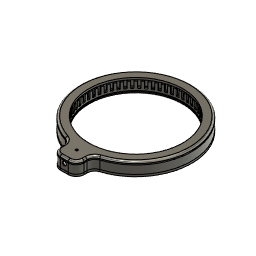
chassis_router (Autodesk Fusion 360 design; units mm, degrees)
Autodesk Fusion 360 part; units mm, degrees
ref_plane "WorkPlane1" through (0, 3.302, 0) normal (0, 1, 0) x (0, 0, 1)
sketch "l1_mirror_base" plane through (0, 0, 0) normal (0, 1, 0) x (1, 0, 0)
  circle A0 centre (0, 0) radius 180.975
  circle A1 centre (0, 0) radius 152.4
  line L0 (0, 0) -> (-90.4875, 156.7289) construction
  line L1 (0, 0) -> (0, 180.975) construction
  circle A2 centre (-84.455, 146.2804) radius 4.445
  line L2 (-84.455, 146.2804) -> (-88.9, 146.2804) construction
  line L3 (-84.455, 146.2804) -> (-80.01, 146.2804) construction
  line L4 (-86.36, 150.2964) -> (-82.55, 150.2964)
  line L5 (86.36, 150.2964) -> (82.55, 150.2964)
  line L6 (84.455, 146.2804) -> (80.01, 146.2804) construction
  circle A3 centre (84.455, 146.2804) radius 4.445
  line L7 (84.455, 146.2804) -> (88.9, 146.2804) construction
  line L8 (0, 0) -> (0, -180.975) construction
  line L9 (-38.1, -176.919) -> (38.1, -176.919)
  line L10 (38.1, -176.919) -> (38.1, -206.129)
  line L11 (12.7, -231.529) -> (-12.7, -231.529)
  line L12 (-38.1, -206.129) -> (-38.1, -176.919)
  arc A4 (12.7, -231.529) -> (38.1, -206.129) centre (12.7, -206.129) ccw
  arc A5 (-38.1, -206.129) -> (-12.7, -231.529) centre (-12.7, -206.129) ccw
  line L13 (34.925, -185.809) -> (34.925, -206.129)
  arc A6 (12.7, -228.354) -> (34.925, -206.129) centre (12.7, -206.129) ccw
  line L14 (12.7, -228.354) -> (-12.7, -228.354)
  arc A7 (-34.925, -206.129) -> (-12.7, -228.354) centre (-12.7, -206.129) ccw
  line L15 (-34.925, -206.129) -> (-34.925, -185.809)
  line L16 (-28.575, -179.459) -> (28.575, -179.459)
  arc A8 (-28.575, -179.459) -> (-34.925, -185.809) centre (-28.575, -185.809) ccw
  arc A9 (34.925, -185.809) -> (28.575, -179.459) centre (28.575, -185.809) ccw
  arc A10 (-38.1, -196.3629) -> (-55.6846, -172.1952) centre (-63.5, -196.3629) ccw
  arc A11 (55.6846, -172.1952) -> (38.1, -196.3629) centre (63.5, -196.3629) ccw
  line L17 (-84.455, 146.2804) -> (-84.455, 150.2964) construction
  line L18 (-82.55, 150.2964) -> (-82.55, 155.3764)
  line L19 (-86.36, 150.2964) -> (-86.36, 155.3764)
  arc A12 (-82.55, 155.3764) -> (-86.36, 155.3764) centre (-84.455, 155.3764) ccw
  line L20 (-82.55, 155.3764) -> (-86.36, 155.3764) construction
  line L21 (86.36, 150.2964) -> (86.36, 155.3764)
  line L22 (82.55, 150.2964) -> (82.55, 155.3764)
  arc A13 (86.36, 155.3764) -> (82.55, 155.3764) centre (84.455, 155.3764) ccw
  line L23 (86.36, 155.3764) -> (82.55, 155.3764)
  point P0 (90.4875, 156.7289)
  point P1 (38.1, -231.529)
  point P2 (-38.1, -231.529)
  dimension "d12" = 361.95
  dimension "d16" = 304.8
  dimension "d85" = 30
  dimension "d91" = 168.91
  dimension "d99" = 8.89
  dimension "d52" = 76.2
  dimension "d54" = 54.61
  dimension "d55" = 25.4
  dimension "d56" = 25.4
  dimension "d58" = 6.35
  dimension "d59" = 3.175
  dimension "d60" = 2.54
  dimension "d61" = 25.4
  dimension "d141" = 3.81
  dimension "d142" = 5.08
  dimension "d143" = 5.08
  constraint coincident A0.centre A1.centre
  constraint coincident A0 L0.end
  constraint coincident A0 L1.end
  constraint vertical L1
  constraint coincident L0 A2.centre
  constraint coincident A2.centre L2.start
  constraint coincident A2 L2.end
  constraint coincident A2 L3.end
  constraint parallel L2 L3
  constraint horizontal L4
  constraint coincident A2 L4.end
  constraint horizontal L2
  constraint symmetric L0.end L1 P0
  constraint symmetric L1 A2 A3
  constraint symmetric L1 A2.centre L6.start
  constraint symmetric L1 L2.end L7.end
  constraint symmetric L1 L3.end L6.end
  constraint symmetric L1 L4.start L5.start
  constraint symmetric L1 L4.end L5.end
  constraint coincident A0 L8.end
  constraint parallel L1 L8
  constraint horizontal L9
  constraint vertical L10
  constraint horizontal L11
  constraint vertical L12
  constraint coincident A0 L9.start
  constraint coincident P1 L10
  constraint coincident P1 L11
  constraint tangent L10 A4
  constraint tangent L11 A4
  constraint coincident P2 L11
  constraint coincident P2 L12
  constraint tangent L11 A5
  constraint tangent L12 A5
  constraint parallel L10 L13
  constraint concentric A4 A6
  constraint parallel L11 L14
  constraint concentric A5 A7
  constraint parallel L12 L15
  constraint parallel L9 L16
  constraint tangent L13 A6
  constraint tangent A6 L14
  constraint tangent L14 A7
  constraint tangent A7 L15
  constraint tangent L16 A8
  constraint tangent L15 A8
  constraint tangent L13 A9
  constraint tangent L16 A9
  constraint equal A8 A9
  constraint tangent A0 A10
  constraint coincident A0 A10.end
  constraint coincident L12 A10.start
  constraint tangent L12 A10
  constraint symmetric L8 A10.end A11.start
  constraint symmetric L8 A10.start A11.end
  constraint symmetric L8 A10 A11
  constraint midpoint L4 L17.end
  constraint perpendicular L4 L17
  constraint perpendicular L4 L18
  constraint perpendicular L4 L19
  constraint equal L18 L19
  constraint coincident A12.centre L20
  constraint perpendicular L5 L21
  constraint perpendicular L5 L22
  constraint equal L21 L22
  constraint coincident A13.centre L23
  measures "d12" diameter of A0
  measures "d16" diameter of A1
  measures "d85" angle of L0 L1
  measures "d91" distance of A0.centre A2.centre
  measures "d99" diameter of A2
  measures "d52" distance of P1 P2
  measures "d54" distance of L9.end P1
  measures "d55" radius of A4
  measures "d56" radius of A5
  measures "d58" radius of A8
  measures "d59" distance of L12 L15
  measures "d60" distance of L9 L16
  measures "d61" radius of A10
  measures "d141" distance of L4.start L4.end
  measures "d142" distance of L4.end L18.end
  measures "d143" distance of L5.end L22.end
extrude "Extrude1" add sketch "l1_mirror_base" along normal up to surface (3.302 mm away) contours A0 L9 | A0 L12 A10 | A0 L10 A11 | A0 L9 L16 | A0 L10 L11 L12 A4 A5 L13 A6 L14 A7 L15 L16 A8 A9 | A0 L16 makes body 1
ref_plane "WorkPlane2" through (0, 6.35, 0) normal (0, 1, 0) x (0, 0, 1)
sketch "l1_mirror" plane through (0, 3.302, 0) normal (0, 1, 0) x (1, 0, 0)
  circle A0 centre (0, 0) radius 180.975
  circle A1 centre (0, 0) radius 163.195
  circle A2 centre (-84.455, 146.2804) radius 4.445
  circle A3 centre (84.455, 146.2804) radius 4.445
  arc A4 (55.6846, -172.1952) -> (-55.6846, -172.1952) centre (0, 0) ccw
  line L0 (-38.1, -196.3629) -> (-38.1, -206.129)
  arc A5 (-38.1, -206.129) -> (-12.7, -231.529) centre (-12.7, -206.129) ccw
  line L1 (-12.7, -231.529) -> (12.7, -231.529)
  arc A6 (12.7, -231.529) -> (38.1, -206.129) centre (12.7, -206.129) ccw
  line L2 (38.1, -206.129) -> (38.1, -196.3629)
  line L3 (-28.575, -179.459) -> (-23.3754, -179.459)
  line L4 (34.925, -185.809) -> (34.925, -206.129)
  arc A7 (12.7, -228.354) -> (34.925, -206.129) centre (12.7, -206.129) ccw
  line L5 (12.7, -228.354) -> (-12.7, -228.354)
  arc A8 (-34.925, -206.129) -> (-12.7, -228.354) centre (-12.7, -206.129) ccw
  line L6 (-34.925, -206.129) -> (-34.925, -185.809)
  arc A9 (-28.575, -179.459) -> (-34.925, -185.809) centre (-28.575, -185.809) ccw
  arc A10 (34.925, -185.809) -> (28.575, -179.459) centre (28.575, -185.809) ccw
  arc A11 (-38.1, -196.3629) -> (-55.6846, -172.1952) centre (-63.5, -196.3629) ccw
  arc A12 (55.6846, -172.1952) -> (38.1, -196.3629) centre (63.5, -196.3629) ccw
  arc A13 (-23.3754, -179.459) -> (23.3754, -179.459) centre (0, 0) ccw
  line L7 (23.3754, -179.459) -> (28.575, -179.459)
  circle A14 centre (0, 0) radius 152.4
  line L8 (-82.55, 155.3764) -> (-82.55, 150.2964)
  arc A15 (-86.36, 150.2964) -> (-82.55, 150.2964) centre (-84.455, 146.2804) ccw
  line L9 (-86.36, 150.2964) -> (-86.36, 155.3764)
  arc A16 (-82.55, 155.3764) -> (-86.36, 155.3764) centre (-84.455, 155.3764) ccw
  line L10 (86.36, 155.3764) -> (86.36, 150.2964)
  arc A17 (82.55, 150.2964) -> (86.36, 150.2964) centre (84.455, 146.2804) ccw
  line L11 (82.55, 150.2964) -> (82.55, 155.3764)
  arc A18 (86.36, 155.3764) -> (82.55, 155.3764) centre (84.455, 155.3764) ccw
  arc A19 (-86.36, 150.2964) -> (-82.55, 150.2964) centre (-84.455, 146.2804) ccw
  line L12 (-82.55, 150.2964) -> (-82.55, 155.3764)
  arc A20 (-82.55, 155.3764) -> (-86.36, 155.3764) centre (-84.455, 155.3764) ccw
  line L13 (-86.36, 155.3764) -> (-86.36, 150.2964)
  arc A21 (82.55, 150.2964) -> (86.36, 150.2964) centre (84.455, 146.2804) ccw
  line L14 (86.36, 150.2964) -> (86.36, 155.3764)
  arc A22 (86.36, 155.3764) -> (82.55, 155.3764) centre (84.455, 155.3764) ccw
  line L15 (82.55, 155.3764) -> (82.55, 150.2964)
  circle A23 centre (0, 0) radius 152.4
  arc A24 (12.7, -228.354) -> (34.925, -206.129) centre (12.7, -206.129) ccw
  line L16 (34.925, -206.129) -> (34.925, -185.809)
  arc A25 (34.925, -185.809) -> (28.575, -179.459) centre (28.575, -185.809) ccw
  line L17 (28.575, -179.459) -> (23.3754, -179.459)
  arc A26 (-23.3754, -179.459) -> (23.3754, -179.459) centre (0, 0) ccw
  line L18 (-23.3754, -179.459) -> (-28.575, -179.459)
  arc A27 (-28.575, -179.459) -> (-34.925, -185.809) centre (-28.575, -185.809) ccw
  line L19 (-34.925, -185.809) -> (-34.925, -206.129)
  arc A28 (-34.925, -206.129) -> (-12.7, -228.354) centre (-12.7, -206.129) ccw
  line L20 (-12.7, -228.354) -> (12.7, -228.354)
  arc A29 (-38.1, -206.129) -> (-12.7, -231.529) centre (-12.7, -206.129) ccw
  line L21 (-38.1, -206.129) -> (-38.1, -196.3629)
  arc A30 (-38.1, -196.3629) -> (-55.6846, -172.1952) centre (-63.5, -196.3629) ccw
  arc A31 (55.6846, -172.1952) -> (-55.6846, -172.1952) centre (0, 0) ccw
  arc A32 (55.6846, -172.1952) -> (38.1, -196.3629) centre (63.5, -196.3629) ccw
  line L22 (38.1, -196.3629) -> (38.1, -206.129)
  arc A33 (12.7, -231.529) -> (38.1, -206.129) centre (12.7, -206.129) ccw
  line L23 (12.7, -231.529) -> (-12.7, -231.529)
  line L24 (84.455, 146.2804) -> (80.01, 146.2804) construction
  line L25 (84.455, 146.2804) -> (88.9, 146.2804) construction
  line L26 (88.9, 146.2804) -> (88.9, 152.8364)
  line L27 (80.01, 146.2804) -> (80.01, 152.8364)
  arc A34 (88.9, 152.8364) -> (80.01, 152.8364) centre (84.455, 152.8364) ccw
  line L28 (-84.455, 146.2804) -> (-88.9, 146.2804) construction
  line L29 (-84.455, 146.2804) -> (-80.01, 146.2804) construction
  line L30 (-80.01, 146.2804) -> (-80.01, 156.0262)
  line L31 (-88.9, 146.2804) -> (-88.9, 156.0262)
  line L32 (84.455, 146.2804) -> (84.455, 157.2814) construction
  line L33 (-84.455, 146.2804) -> (-84.455, 157.2814) construction
  circle A35 centre (-84.455, 152.8364) radius 4.445
  dimension "d18" = 361.95
  dimension "d19" = 326.39
  constraint coincident A0.centre A1.centre
  constraint coincident A3.centre A17.centre
  constraint coincident A21 L24.end
  constraint coincident A21 L25.end
  constraint tangent A21 L26
  constraint tangent A21 L27
  constraint tangent L27 A34
  constraint tangent L26 A34
  constraint coincident A2.centre A15.centre
  constraint coincident A19 L28.end
  constraint coincident A19 L29.end
  constraint tangent A15 L30
  constraint perpendicular L29 L30
  constraint tangent A2 L31
  constraint perpendicular L28 L31
  constraint midpoint A22 L32.end
  constraint perpendicular L24 L32
  constraint perpendicular L25 L32
  constraint tangent A22 A34
  constraint midpoint A16 L33.end
  constraint perpendicular L28 L33
  constraint perpendicular L29 L33
  constraint tangent A20 A35
  constraint tangent L30 A35
  constraint equal L30 L31
  constraint tangent L31 A35
  measures "d18" diameter of A0
  measures "d19" diameter of A1
extrude "Extrude2" add sketch "l1_mirror" along normal up to surface (3.048 mm away) contours A0 A4 A13 A26 A31 | A0 L0 A5 L1 A6 L2 L3 L4 A7 L5 A8 L6 A9 A10 A11 A12 L7 A24 L16 A25 L17 L18 A27 L19 A28 L20 A29 L21 A30 A32 L22 A33 L23 bodies 1
ref_plane "WorkPlane3" through (0, 14.097, 0) normal (0, 1, 0) x (0, 0, 1)
sketch "l2_led_base" plane through (0, 6.35, 0) normal (0, 1, 0) x (1, 0, 0)
  circle A0 centre (0, 0) radius 180.975
  circle A1 centre (0, 0) radius 152.4
  line L0 (0, 0) -> (-9.4715, 180.727) construction
  line L1 (0, 0) -> (0, 180.975) construction
  arc A2 (55.6846, -172.1952) -> (-55.6846, -172.1952) centre (0, 0) ccw
  arc A3 (-38.1, -196.3629) -> (-55.6846, -172.1952) centre (-63.5, -196.3629) ccw
  line L2 (-38.1, -196.3629) -> (-38.1, -206.129)
  arc A4 (-38.1, -206.129) -> (-12.7, -231.529) centre (-12.7, -206.129) ccw
  line L3 (-12.7, -231.529) -> (12.7, -231.529)
  arc A5 (12.7, -231.529) -> (38.1, -206.129) centre (12.7, -206.129) ccw
  line L4 (38.1, -206.129) -> (38.1, -196.3629)
  arc A6 (55.6846, -172.1952) -> (38.1, -196.3629) centre (63.5, -196.3629) ccw
  line L5 (88.9, 152.8364) -> (88.9, 146.2804)
  arc A7 (80.01, 146.2804) -> (88.9, 146.2804) centre (84.455, 146.2804) ccw
  line L6 (80.01, 146.2804) -> (80.01, 152.8364)
  arc A8 (88.9, 152.8364) -> (80.01, 152.8364) centre (84.455, 152.8364) ccw
  arc A9 (-28.575, -179.459) -> (-34.925, -185.809) centre (-28.575, -185.809) ccw
  line L7 (-28.575, -179.459) -> (-23.3754, -179.459)
  arc A10 (-23.3754, -179.459) -> (23.3754, -179.459) centre (0, 0) ccw
  line L8 (23.3754, -179.459) -> (28.575, -179.459)
  arc A11 (34.925, -185.809) -> (28.575, -179.459) centre (28.575, -185.809) ccw
  line L9 (34.925, -185.809) -> (34.925, -206.129)
  arc A12 (12.7, -228.354) -> (34.925, -206.129) centre (12.7, -206.129) ccw
  line L10 (12.7, -228.354) -> (-12.7, -228.354)
  arc A13 (-34.925, -206.129) -> (-12.7, -228.354) centre (-12.7, -206.129) ccw
  line L11 (-34.925, -206.129) -> (-34.925, -185.809)
  line L12 (-80.01, 152.8364) -> (-80.01, 146.2804)
  arc A14 (-88.9, 146.2804) -> (-80.01, 146.2804) centre (-84.455, 146.2804) ccw
  line L13 (-88.9, 146.2804) -> (-88.9, 152.8364)
  arc A15 (-80.01, 152.8364) -> (-88.9, 152.8364) centre (-84.455, 152.8364) ccw
  circle A16 centre (0, 0) radius 163.195
  dimension "d23" = 361.95
  dimension "d24" = 304.8
  dimension "d1" = 3
  constraint coincident A0.centre A1.centre
  constraint coincident A0 L0.end
  constraint coincident A0 L1.end
  constraint vertical L1
  measures "d23" diameter of A0
  measures "d24" diameter of A1
  measures "d1" angle of L0 L1
extrude "Extrude3" add sketch "l2_led_base" along normal up to surface (7.747 mm away) separate body contours A0 A2 A10 | A0 A3 L2 A4 L3 A5 L4 A6 A9 L7 L8 A11 L9 A12 L10 A13 L11 | L5 A7 L6 A8 | L12 A14 L13 A15 | A16 makes body 2
ref_plane "WorkPlane4" through (0, 32.8422, 0) normal (0, 1, 0) x (0, 0, 1)
sketch "l2_leds" plane through (0, 14.097, 0) normal (0, 1, 0) x (1, 0, 0)
  circle A0 centre (0, 0) radius 180.975
  circle A1 centre (0, 0) radius 159.639
  line L0 (0, 0) -> (0, 180.975) construction
  circle A2 centre (0, 0) radius 152.4 construction
  line L1 (0, 0) -> (-7.976, 152.1911) construction
  line L2 (0, 0) -> (-11.9572, 151.9302) construction
  line L3 (0, 0) -> (-3.9894, 152.3478) construction
  arc A3 (-3.9894, 152.3478) -> (-11.9572, 151.9302) centre (0, 0) ccw
  circle A4 centre (0, 0) radius 157.099
  line L4 (-3.9894, 152.3478) -> (4.1124, -157.0452)
  line L5 (-11.9572, 151.9302) -> (12.3258, -156.6147)
  line L6 (-3.9894, 152.3478) -> (-4.1124, 157.0452)
  line L7 (-11.9572, 151.9302) -> (-12.3258, 156.6147)
  arc A5 (55.6846, -172.1952) -> (38.1, -196.3629) centre (63.5, -196.3629) ccw
  arc A6 (-38.1, -196.3629) -> (-55.6846, -172.1952) centre (-63.5, -196.3629) ccw
  line L8 (-38.1, -196.3629) -> (-38.1, -206.129)
  arc A7 (-38.1, -206.129) -> (-12.7, -231.529) centre (-12.7, -206.129) ccw
  line L9 (-12.7, -231.529) -> (12.7, -231.529)
  arc A8 (12.7, -231.529) -> (38.1, -206.129) centre (12.7, -206.129) ccw
  line L10 (38.1, -206.129) -> (38.1, -196.3629)
  line L11 (0, 0) -> (0, -171.45) construction
  line L12 (6.35, -159.5127) -> (6.35, -180.8636)
  line L13 (-6.35, -180.8636) -> (-6.35, -159.5127)
  arc A9 (9.3393, -159.3656) -> (6.35, -162.5351) centre (9.525, -162.5351) ccw
  arc A10 (-6.35, -162.5351) -> (-9.3393, -159.3656) centre (-9.525, -162.5351) ccw
  circle A11 centre (0, 0) radius 152.4
  arc A12 (55.6846, -172.1952) -> (-55.6846, -172.1952) centre (0, 0) ccw
  arc A13 (55.6846, -172.1952) -> (38.1, -196.3629) centre (63.5, -196.3629) ccw
  arc A14 (55.6846, -172.1952) -> (-55.6846, -172.1952) centre (0, 0) ccw
  arc A15 (-38.1, -196.3629) -> (-55.6846, -172.1952) centre (-63.5, -196.3629) ccw
  line L14 (-38.1, -196.3629) -> (-38.1, -206.129)
  arc A16 (-38.1, -206.129) -> (-12.7, -231.529) centre (-12.7, -206.129) ccw
  line L15 (-12.7, -231.529) -> (12.7, -231.529)
  arc A17 (12.7, -231.529) -> (38.1, -206.129) centre (12.7, -206.129) ccw
  line L16 (38.1, -206.129) -> (38.1, -196.3629)
  line L17 (88.9, 152.8364) -> (88.9, 146.2804)
  arc A18 (80.01, 146.2804) -> (88.9, 146.2804) centre (84.455, 146.2804) ccw
  line L18 (80.01, 146.2804) -> (80.01, 152.8364)
  arc A19 (88.9, 152.8364) -> (80.01, 152.8364) centre (84.455, 152.8364) ccw
  arc A20 (-28.575, -179.459) -> (-34.925, -185.809) centre (-28.575, -185.809) ccw
  line L19 (-28.575, -179.459) -> (-23.3754, -179.459)
  arc A21 (-23.3754, -179.459) -> (23.3754, -179.459) centre (0, 0) ccw
  line L20 (23.3754, -179.459) -> (28.575, -179.459)
  arc A22 (34.925, -185.809) -> (28.575, -179.459) centre (28.575, -185.809) ccw
  line L21 (34.925, -185.809) -> (34.925, -206.129)
  arc A23 (12.7, -228.354) -> (34.925, -206.129) centre (12.7, -206.129) ccw
  line L22 (12.7, -228.354) -> (-12.7, -228.354)
  arc A24 (-34.925, -206.129) -> (-12.7, -228.354) centre (-12.7, -206.129) ccw
  line L23 (-34.925, -206.129) -> (-34.925, -185.809)
  line L24 (-80.01, 152.8364) -> (-80.01, 146.2804)
  arc A25 (-88.9, 146.2804) -> (-80.01, 146.2804) centre (-84.455, 146.2804) ccw
  line L25 (-88.9, 146.2804) -> (-88.9, 152.8364)
  arc A26 (-80.01, 152.8364) -> (-88.9, 152.8364) centre (-84.455, 152.8364) ccw
  circle A27 centre (0, 0) radius 163.195
  line L26 (34.925, -185.809) -> (34.925, -206.129)
  arc A28 (12.7, -228.354) -> (34.925, -206.129) centre (12.7, -206.129) ccw
  line L27 (12.7, -228.354) -> (-12.7, -228.354)
  arc A29 (-34.925, -206.129) -> (-12.7, -228.354) centre (-12.7, -206.129) ccw
  line L28 (-34.925, -206.129) -> (-34.925, -185.809)
  arc A30 (-28.575, -179.459) -> (-34.925, -185.809) centre (-28.575, -185.809) ccw
  line L29 (-28.575, -179.459) -> (-23.3754, -179.459)
  arc A31 (-23.3754, -179.459) -> (23.3754, -179.459) centre (0, 0) ccw
  line L30 (23.3754, -179.459) -> (28.575, -179.459)
  arc A32 (34.925, -185.809) -> (28.575, -179.459) centre (28.575, -185.809) ccw
  dimension "d28" = 361.95
  dimension "d29" = 319.278
  dimension "d6" = 304.8
  dimension "d7" = 3
  dimension "d8" = 3
  dimension "d10" = 314.198
  dimension "d100" = 12.7
  dimension "d101" = 3.175
  constraint coincident A0.centre A1.centre
  constraint concentric A0 A1
  constraint coincident A0 L0.end
  constraint vertical L0
  constraint coincident A2 L1.end
  constraint coincident A2 L2.end
  constraint coincident A2 L3.end
  constraint symmetric L1 L2 L3
  constraint concentric A2 A3
  constraint concentric A2 A4
  constraint coincident A4 L4.end
  constraint parallel L3 L4
  constraint coincident A4 L5.end
  constraint parallel L2 L5
  constraint coincident A4 L6.end
  constraint parallel L4 L6
  constraint coincident A4 L7.end
  constraint parallel L5 L7
  constraint coincident A1 L12.start
  constraint coincident A1 L13.end
  constraint vertical L13
  constraint vertical L12
  constraint symmetric L11 L12 L13
  constraint tangent A1 A9
  constraint coincident A1 A9.start
  constraint coincident L12 A9.end
  constraint tangent L12 A9
  constraint symmetric L11 A9.end A10.start
  constraint symmetric L11 A9.start A10.end
  constraint symmetric L11 A9 A10
  constraint coincident A0 L12.end
  constraint coincident A0 L13.start
  measures "d28" diameter of A0
  measures "d29" diameter of A1
  measures "d6" diameter of A2
  measures "d7" angle of L0 L1
  measures "d8" angle of L2 L3
  measures "d10" diameter of A4
  measures "d100" distance of L12 L13
  measures "d101" radius of A9
extrude "Extrude4" add sketch "l2_leds" along normal up to surface (18.7452 mm away) contours A0 L12 L13 A12 A14 A21 A27 A31 | A0 A5 A6 L8 A7 L9 A8 L10 A13 A15 L14 A16 L15 A17 L16 A20 L19 L20 A22 L21 A23 L22 A24 L23 L26 A28 L27 A29 L28 A30 L29 L30 A32 | A1 L12 L13 A9 A10 A27 | L17 A18 L18 A19 | L24 A25 L25 A26 bodies 2
sketch "l3_cap_base" plane through (0, 32.8422, 0) normal (0, 1, 0) x (1, 0, 0)
  circle A0 centre (0, 0) radius 180.975
  circle A1 centre (0, 0) radius 163.195
  arc A2 (-23.3754, -179.459) -> (-6.35, -180.8636) centre (0, 0) ccw
  arc A3 (-38.1, -196.3629) -> (-55.6846, -172.1952) centre (-63.5, -196.3629) ccw
  line L0 (-38.1, -196.3629) -> (-38.1, -206.129)
  arc A4 (-38.1, -206.129) -> (-12.7, -231.529) centre (-12.7, -206.129) ccw
  line L1 (-12.7, -231.529) -> (12.7, -231.529)
  arc A5 (12.7, -231.529) -> (38.1, -206.129) centre (12.7, -206.129) ccw
  line L2 (38.1, -206.129) -> (38.1, -196.3629)
  arc A6 (55.6846, -172.1952) -> (38.1, -196.3629) centre (63.5, -196.3629) ccw
  line L3 (6.35, -162.5351) -> (6.35, -180.8636)
  line L4 (-6.35, -180.8636) -> (-6.35, -162.5351)
  arc A7 (-6.35, -162.5351) -> (-9.3393, -159.3656) centre (-9.525, -162.5351) ccw
  arc A8 (9.3393, -159.3656) -> (-9.3393, -159.3656) centre (0, 0) ccw
  arc A9 (9.3393, -159.3656) -> (6.35, -162.5351) centre (9.525, -162.5351) ccw
  line L5 (34.925, -185.809) -> (34.925, -206.129)
  arc A10 (12.7, -228.354) -> (34.925, -206.129) centre (12.7, -206.129) ccw
  line L6 (12.7, -228.354) -> (-12.7, -228.354)
  arc A11 (-34.925, -206.129) -> (-12.7, -228.354) centre (-12.7, -206.129) ccw
  line L7 (-34.925, -206.129) -> (-34.925, -185.809)
  arc A12 (-28.575, -179.459) -> (-34.925, -185.809) centre (-28.575, -185.809) ccw
  line L8 (-28.575, -179.459) -> (-23.3754, -179.459)
  arc A13 (6.35, -180.8636) -> (23.3754, -179.459) centre (0, 0) ccw
  line L9 (23.3754, -179.459) -> (28.575, -179.459)
  arc A14 (34.925, -185.809) -> (28.575, -179.459) centre (28.575, -185.809) ccw
  arc A15 (55.6846, -172.1952) -> (-55.6846, -172.1952) centre (0, 0) ccw
  dimension "d33" = 361.95
  dimension "d34" = 326.39
  constraint coincident A0.centre A1.centre
  measures "d33" diameter of A0
  measures "d34" diameter of A1
ref_plane "WorkPlane5" through (0, 36.6522, 0) normal (0, 1, 0) x (0, 0, 1)
extrude "Extrude5" add sketch "l3_cap_base" along normal up to surface (3.81 mm away) separate body contours A0 A1 A2 L3 L4 A13 A15 | A0 A3 L0 A4 L1 A5 L2 A6 L5 A10 L6 A11 L7 A12 L8 L9 A14 | A0 A2 L5 A10 L6 A11 L7 A12 L8 A13 L9 A14 | A0 A1 L3 L4 makes body 3
ref_plane "WorkPlane7" through (0, 43.0022, 0) normal (0, 1, 0) x (0, 0, 1)
sketch "l3_cap" plane through (0, 36.6522, 0) normal (0, 1, 0) x (1, 0, 0)
  circle A0 centre (0, 0) radius 180.975
  circle A1 centre (0, 0) radius 152.4
  arc A2 (-38.1, -196.3629) -> (-55.6846, -172.1952) centre (-63.5, -196.3629) ccw
  line L0 (-38.1, -196.3629) -> (-38.1, -206.129)
  arc A3 (-38.1, -206.129) -> (-12.7, -231.529) centre (-12.7, -206.129) ccw
  line L1 (-12.7, -231.529) -> (12.7, -231.529)
  arc A4 (12.7, -231.529) -> (38.1, -206.129) centre (12.7, -206.129) ccw
  line L2 (38.1, -206.129) -> (38.1, -196.3629)
  arc A5 (55.6846, -172.1952) -> (38.1, -196.3629) centre (63.5, -196.3629) ccw
  arc A6 (55.6846, -172.1952) -> (-55.6846, -172.1952) centre (0, 0) ccw
  circle A7 centre (0, 0) radius 163.195
  dimension "d43" = 361.95
  dimension "d44" = 304.8
  constraint coincident A0.centre A1.centre
  measures "d43" diameter of A0
  measures "d44" diameter of A1
extrude "Extrude7" add sketch "l3_cap" along normal up to surface (6.35 mm away) contours A0 A6 | A0 A2 L0 A3 L1 A4 L2 A5 | A7 bodies 3
ref_plane "WorkPlane8" through (0, 39.8272, 0) normal (0, -1, 0) x (-1, 0, 0)
extrude "Extrude10" add sketch "l2_leds" along normal up to surface (18.7452 mm away) contours A3 A4 L6 L7 A11 bodies 2
sketch "Circuit case lid" plane through (0, 39.8272, 0) normal (0, -1, 0) x (1, 0, 0)
  arc A0 (55.5625, -168.8954) -> (38.1, -193.0233) centre (63.5, -193.0233) ccw
  arc A1 (55.5625, -168.8954) -> (-55.5625, -168.8954) centre (0, 0) ccw
  arc A2 (-38.1, -193.0233) -> (-55.5625, -168.8954) centre (-63.5, -193.0233) ccw
  line L0 (-38.1, -193.0233) -> (-38.1, -202.8799)
  arc A3 (-38.1, -202.8799) -> (-12.7, -228.2799) centre (-12.7, -202.8799) ccw
  line L1 (-12.7, -228.2799) -> (12.7, -228.2799)
  arc A4 (12.7, -228.2799) -> (38.1, -202.8799) centre (12.7, -202.8799) ccw
  line L2 (38.1, -202.8799) -> (38.1, -193.0233)
  arc A5 (34.925, 206.129) -> (12.7, 228.354) centre (12.7, 206.129) ccw
  line L3 (34.925, 206.129) -> (34.925, 185.809)
  arc A6 (28.575, 179.459) -> (34.925, 185.809) centre (28.575, 185.809) ccw
  line L4 (28.575, 179.459) -> (23.3754, 179.459)
  arc A7 (23.3754, 179.459) -> (-23.3754, 179.459) centre (0, 0) ccw
  line L5 (-23.3754, 179.459) -> (-28.575, 179.459)
  arc A8 (-34.925, 185.809) -> (-28.575, 179.459) centre (-28.575, 185.809) ccw
  line L6 (-34.925, 185.809) -> (-34.925, 206.129)
  arc A9 (-12.7, 228.354) -> (-34.925, 206.129) centre (-12.7, 206.129) ccw
  line L7 (-12.7, 228.354) -> (12.7, 228.354)
  arc A10 (-55.6846, 172.1952) -> (55.6846, 172.1952) centre (0, 0) ccw
  arc A11 (38.1, 196.3629) -> (55.6846, 172.1952) centre (63.5, 196.3629) ccw
  line L8 (38.1, 196.3629) -> (38.1, 206.129)
  arc A12 (38.1, 206.129) -> (12.7, 231.529) centre (12.7, 206.129) ccw
  line L9 (12.7, 231.529) -> (-12.7, 231.529)
  arc A13 (-12.7, 231.529) -> (-38.1, 206.129) centre (-12.7, 206.129) ccw
  line L10 (-38.1, 206.129) -> (-38.1, 196.3629)
  arc A14 (-55.6846, 172.1952) -> (-38.1, 196.3629) centre (-63.5, 196.3629) ccw
  circle A15 centre (0, 0) radius 152.4
  arc A16 (-82.55, -150.2964) -> (-86.36, -150.2964) centre (-84.455, -146.2804) ccw
  line L11 (-82.55, -150.2964) -> (-82.55, -155.3764)
  arc A17 (-86.36, -155.3764) -> (-82.55, -155.3764) centre (-84.455, -155.3764) ccw
  line L12 (-86.36, -155.3764) -> (-86.36, -150.2964)
  arc A18 (86.36, -150.2964) -> (82.55, -150.2964) centre (84.455, -146.2804) ccw
  line L13 (86.36, -150.2964) -> (86.36, -155.3764)
  arc A19 (82.55, -155.3764) -> (86.36, -155.3764) centre (84.455, -155.3764) ccw
  line L14 (82.55, -155.3764) -> (82.55, -150.2964)
extrude "Extrude11" cut sketch "Circuit case lid" along normal up to surface (33.4772 mm away) contours A5 L3 A6 L4 A7 L5 A8 L6 A9 L7 bodies 2 3
sketch "pcb_locator" plane through (0, 32.8422, 0) normal (0, -1, 0) x (1, 0, 0)
  line L0 (34.925, 206.129) -> (34.925, 185.809)
  arc A0 (28.575, 179.459) -> (34.925, 185.809) centre (28.575, 185.809) ccw
  line L1 (28.575, 179.459) -> (23.3754, 179.459)
  arc A1 (23.3754, 179.459) -> (-23.3754, 179.459) centre (0, 0) ccw
  line L2 (-23.3754, 179.459) -> (-28.575, 179.459)
  arc A2 (-34.925, 185.809) -> (-28.575, 179.459) centre (-28.575, 185.809) ccw
  line L3 (-34.925, 185.809) -> (-34.925, 206.129)
  arc A3 (-12.7, 228.354) -> (-34.925, 206.129) centre (-12.7, 206.129) ccw
  line L4 (-12.7, 228.354) -> (12.7, 228.354)
  arc A4 (34.925, 206.129) -> (12.7, 228.354) centre (12.7, 206.129) ccw
  line L5 (-38.1, 206.129) -> (-38.1, 196.3629)
  arc A5 (-55.6846, 172.1952) -> (-38.1, 196.3629) centre (-63.5, 196.3629) ccw
  arc A6 (-55.6846, 172.1952) -> (55.6846, 172.1952) centre (0, 0) ccw
  arc A7 (38.1, 196.3629) -> (55.6846, 172.1952) centre (63.5, 196.3629) ccw
  line L6 (38.1, 196.3629) -> (38.1, 206.129)
  arc A8 (38.1, 206.129) -> (12.7, 231.529) centre (12.7, 206.129) ccw
  line L7 (12.7, 231.529) -> (-12.7, 231.529)
  arc A9 (-12.7, 231.529) -> (-38.1, 206.129) centre (-12.7, 206.129) ccw
  arc A10 (-12.7, 226.7538) -> (-33.3248, 206.129) centre (-12.7, 206.129) ccw
  line L8 (-33.3248, 185.809) -> (-33.3248, 206.129)
  arc A11 (-33.3248, 185.809) -> (-28.575, 181.0592) centre (-28.575, 185.809) ccw
  line L9 (-23.479, 181.0592) -> (-28.575, 181.0592)
  arc A12 (23.479, 181.0592) -> (-23.479, 181.0592) centre (0, 0) ccw
  line L10 (28.575, 181.0592) -> (23.479, 181.0592)
  arc A13 (28.575, 181.0592) -> (33.3248, 185.809) centre (28.575, 185.809) ccw
  line L11 (33.3248, 206.129) -> (33.3248, 185.809)
  arc A14 (33.3248, 206.129) -> (12.7, 226.7538) centre (12.7, 206.129) ccw
  line L12 (-12.7, 226.7538) -> (12.7, 226.7538)
  circle A15 centre (0, 0) radius 163.195
  dimension "d137" = 1.6002
pattern_circular "C-Pattern1" count 60 over 360 about axis through (0, 1.75, 0) along (0, 1, 0) of "Extrude10"
chamfer "Chamfer1" distance 1.905 angle 45 60 edges at (0, 14.097, -152.4) (15.9301, 14.097, -151.5651) (31.6857, 14.097, -149.0697) (47.0942, 14.097, -144.941) (61.9867, 14.097, -139.2243) (76.2, 14.097, -131.9823) (89.5785, 14.097, -123.2942) (113.2553, 14.097, -101.9755) (101.9755, 14.097, -113.2553) (123.2942, 14.097, -89.5785) (131.9823, 14.097, -76.2) (139.2243, 14.097, -61.9867) (144.941, 14.097, -47.0942) (151.5651, 14.097, -15.9301) (152.4, 14.097, 0) (149.0697, 14.097, -31.6857) (151.5651, 14.097, 15.9301) (149.0697, 14.097, 31.6857) (144.941, 14.097, 47.0942) (139.2243, 14.097, 61.9867) (131.9823, 14.097, 76.2) (123.2942, 14.097, 89.5785) (113.2553, 14.097, 101.9755) (101.9755, 14.097, 113.2553) (89.5785, 14.097, 123.2942) (76.2, 14.097, 131.9823) (61.9867, 14.097, 139.2243) (47.0942, 14.097, 144.941) (31.6857, 14.097, 149.0697) (15.9301, 14.097, 151.5651) (0, 14.097, 152.4) (-15.9301, 14.097, 151.5651) (-31.6857, 14.097, 149.0697) (-47.0942, 14.097, 144.941) (-61.9867, 14.097, 139.2243) (-76.2, 14.097, 131.9823) (-89.5785, 14.097, 123.2942) (-101.9755, 14.097, 113.2553) (-113.2553, 14.097, 101.9755) (-123.2942, 14.097, 89.5785) (-131.9823, 14.097, 76.2) (-139.2243, 14.097, 61.9867) (-144.941, 14.097, 47.0942) (-149.0697, 14.097, 31.6857) (-151.5651, 14.097, 15.9301) (-152.4, 14.097, 0) (-151.5651, 14.097, -15.9301) (-149.0697, 14.097, -31.6857) (-144.941, 14.097, -47.0942) (-139.2243, 14.097, -61.9867) (-131.9823, 14.097, -76.2) (-123.2942, 14.097, -89.5785) (-113.2553, 14.097, -101.9755) (-101.9755, 14.097, -113.2553) (-89.5785, 14.097, -123.2942) (-31.6857, 14.097, -149.0697) (-15.9301, 14.097, -151.5651) (-47.0942, 14.097, -144.941) (-61.9867, 14.097, -139.2243) (-76.2, 14.097, -131.9823) on bodies 2
sketch "PCB_Holes_cap" plane through (0, 32.8422, 0) normal (0, -1, 0) x (1, 0, 0)
  line L0 (0, 185.6252) -> (0, 197.0252) construction
  circle A0 centre (0, 191.3252) radius 3.81
  circle A1 centre (24.5, 209.5752) radius 3.302
  circle A2 centre (24.5, 209.5752) radius 0.5953
  line L1 (34.925, 206.129) -> (34.925, 185.809)
  arc A3 (28.575, 179.459) -> (34.925, 185.809) centre (28.575, 185.809) ccw
  line L2 (28.575, 179.459) -> (23.3754, 179.459)
  arc A4 (23.3754, 179.459) -> (-23.3754, 179.459) centre (0, 0) ccw
  line L3 (-23.3754, 179.459) -> (-28.575, 179.459)
  arc A5 (-34.925, 185.809) -> (-28.575, 179.459) centre (-28.575, 185.809) ccw
  line L4 (-34.925, 185.809) -> (-34.925, 206.129)
  arc A6 (-12.7, 228.354) -> (-34.925, 206.129) centre (-12.7, 206.129) ccw
  line L5 (-12.7, 228.354) -> (12.7, 228.354)
  arc A7 (34.925, 206.129) -> (12.7, 228.354) centre (12.7, 206.129) ccw
  line L6 (-38.1, 206.129) -> (-38.1, 196.3629)
  arc A8 (-55.6846, 172.1952) -> (-38.1, 196.3629) centre (-63.5, 196.3629) ccw
  arc A9 (-55.6846, 172.1952) -> (55.6846, 172.1952) centre (0, 0) ccw
  arc A10 (38.1, 196.3629) -> (55.6846, 172.1952) centre (63.5, 196.3629) ccw
  line L7 (38.1, 196.3629) -> (38.1, 206.129)
  arc A11 (38.1, 206.129) -> (12.7, 231.529) centre (12.7, 206.129) ccw
  line L8 (12.7, 231.529) -> (-12.7, 231.529)
  arc A12 (-12.7, 231.529) -> (-38.1, 206.129) centre (-12.7, 206.129) ccw
  circle A13 centre (0, 185.6252) radius 1.3
  circle A14 centre (0, 197.0252) radius 1.3
  circle A15 centre (-24.5, 209.5752) radius 1.5
  circle A16 centre (-24.5, 186.5752) radius 1.5
  circle A17 centre (24.5, 209.5752) radius 1.5
  circle A18 centre (24.5, 186.5752) radius 1.5
  circle A19 centre (0, 210.8752) radius 0.65
  circle A20 centre (18.88, 202.8952) radius 0.175
  circle A21 centre (7.5, 193.8252) radius 0.5
  circle A22 centre (9.03, 185.6394) radius 0.175
  circle A23 centre (13.42, 186.8252) radius 0.508
  circle A24 centre (0.5, 191.5752) radius 0.175
  circle A25 centre (7.5, 188.8252) radius 0.5
  circle A26 centre (10.4, 197.2352) radius 0.175
  circle A27 centre (-4.8, 213.8752) radius 0.65
  circle A28 centre (10.5, 204.5752) radius 0.175
  circle A29 centre (-20.34, 187.1352) radius 0.508
  circle A30 centre (-21.61, 192.6552) radius 0.3
  circle A31 centre (15.96, 186.8252) radius 0.508
  circle A32 centre (-7.08, 196.1152) radius 0.175
  circle A33 centre (7.5, 191.3252) radius 0.5
  circle A34 centre (8.32, 197.2152) radius 0.175
  circle A35 centre (0, 216.6752) radius 0.65
  circle A36 centre (-7, 188.8252) radius 0.5
  circle A37 centre (10.88, 186.8252) radius 0.508
  circle A38 centre (-13.44, 200.5352) radius 0.175
  circle A39 centre (-7, 193.8252) radius 0.5
  circle A40 centre (18.5, 186.8252) radius 0.508
  circle A41 centre (-17.61, 192.6552) radius 0.3
  circle A42 centre (-20.34, 189.6752) radius 0.508
  circle A43 centre (-19.61, 192.6552) radius 0.3
  line L9 (27.5, 220.5752) -> (27.5, 182.5752)
  line L10 (27.5, 182.5752) -> (-27.5, 182.5752)
  line L11 (-27.5, 182.5752) -> (-27.5, 220.5752)
  line L12 (-27.5, 220.5752) -> (27.5, 220.5752)
  line L13 (24.5, 212.8772) -> (24.5, 206.2732) construction
  circle A44 centre (0, 0) radius 163.195
  circle A45 centre (-24.5, 209.5752) radius 0.5953
  circle A46 centre (-24.5, 209.5752) radius 3.302
  circle A47 centre (-24.5, 186.5752) radius 0.5953
  circle A48 centre (-24.5, 186.5752) radius 3.302
  circle A49 centre (24.5, 186.5752) radius 0.5953
  circle A50 centre (24.5, 186.5752) radius 3.302
  line L14 (-24.5, 186.5752) -> (-21.198, 186.5752) construction
  line L15 (-24.5, 186.5752) -> (-24.5, 189.8772) construction
  line L16 (-24.5, 209.5752) -> (-24.5, 206.2732) construction
  line L17 (-24.5, 209.5752) -> (-24.5, 212.8772) construction
  line L18 (24.5, 186.5752) -> (21.198, 186.5752) construction
  line L19 (24.5, 186.5752) -> (24.5, 189.8772) construction
  arc A51 (-34.925, 200.3022) -> (-24.5, 189.8772) centre (-24.5, 200.3022) ccw
  arc A52 (-24.5, 206.2732) -> (-34.925, 200.3022) centre (-28.0025, 200.3022) ccw
  arc A53 (-21.198, 186.5752) -> (-14.4992, 180.3932) centre (-14.9961, 186.5752) ccw
  arc A54 (14.4992, 180.3932) -> (21.198, 186.5752) centre (14.9961, 186.5752) ccw
  arc A55 (24.5, 189.8772) -> (34.925, 200.3022) centre (24.5, 200.3022) ccw
  arc A56 (34.925, 200.3022) -> (24.5, 206.2732) centre (28.0025, 200.3022) ccw
  arc A57 (24.5, 212.8772) -> (28.2277, 222.03) centre (24.5, 218.2127) ccw
  arc A58 (-28.2277, 222.03) -> (-24.5, 212.8772) centre (-24.5, 218.2127) ccw
  dimension "d67" = 7.62
  dimension "d72" = 6.604
  dimension "d124" = 1.1906
  constraint coincident L0 A0.centre
  constraint midpoint L0 A0.centre
  constraint concentric A2 A17
  constraint concentric A1 A17
  constraint coincident L0.start A13.centre
  constraint coincident L0.end A14.centre
  constraint coincident A1 L13.start
  constraint coincident A1 L13.end
  constraint vertical L13
  constraint coincident A1.centre L13
  constraint concentric A15 A45
  constraint concentric A15 A46
  constraint concentric A16 A47
  constraint concentric A16 A48
  constraint concentric A18 A49
  constraint concentric A49 A50
  constraint equal A1 A50
  constraint equal A2 A49
  constraint equal A47 A49
  constraint equal A45 A47
  constraint equal A46 A48
  constraint equal A1 A46
  constraint coincident A16.centre A47.centre
  constraint coincident A48 L14.end
  constraint horizontal L14
  constraint coincident A48 L15.end
  constraint perpendicular L14 L15
  constraint coincident A15.centre A45.centre
  constraint coincident A46 L16.end
  constraint parallel L15 L16
  constraint coincident A46 L17.end
  constraint parallel L16 L17
  constraint coincident A18.centre A49.centre
  constraint coincident A50 L18.end
  constraint horizontal L18
  constraint coincident A50 L19.end
  constraint perpendicular L18 L19
  constraint tangent A48 A51
  constraint coincident L4 A51.start
  constraint coincident A51.start A52.end
  constraint tangent L4 A51
  constraint tangent L4 A52
  constraint coincident A4 A53.end
  constraint tangent A48 A53
  constraint tangent A4 A53
  constraint tangent A50 A54
  constraint coincident A4 A54.start
  constraint tangent A4 A54
  constraint coincident L1 A55.end
  constraint tangent L1 A55
  constraint tangent L1 A56
  constraint coincident A55.end A56.start
  constraint coincident A7 A57.end
  constraint tangent A1 A57
  constraint tangent A7 A57
  constraint tangent A46 A58
  constraint coincident A6 A58.start
  constraint tangent A6 A58
  constraint tangent A50 A55
  measures "d67" diameter of A0
  measures "d72" diameter of A1
  measures "d124" diameter of A2
extrude "Extrude12" cut sketch "PCB_Holes_cap" against normal up to surface (10.16 mm away) contours A0 | A24 bodies 3
extrude "Extrude13" add sketch "PCB_Holes_cap" against normal up to surface (6.985 mm away) contours A1 L9 A56 | A1 L9 A57 | A1 A56 | A1 L1 A7 L9 A56 A57 | A1 L9 | A1 L9 A56 | L1 A3 L2 A4 L9 L10 A50 A54 A55 | L9 A50 A55 | L11 A46 A58 | L4 A6 L11 A46 A52 A58 | L9 A50 | L9 A50 | L11 A46 A52 | L11 A46 | L9 L10 A50 A54 | L11 A46 A52 | A46 A52 | A4 L3 A5 L4 L10 L11 A48 A51 A53 | L10 L11 A48 A53 | L11 A48 A51 | L11 A48 | L11 A48 | A15 | A16 | A17 | A18 bodies 3
fillet "Fillet1" radius 6.35 8 edges at (0, 43.0022, -180.975) (42.9614, 43.0022, 181.4189) (38.1, 43.0022, 201.246) (30.6605, 43.0022, 224.0895) (0, 43.0022, 231.529) (-30.6605, 43.0022, 224.0895) (-38.1, 43.0022, 201.246) (-42.9614, 43.0022, 181.4189) on bodies 3
fillet "Fillet5" radius 2.54 16 edges at (-21.0831, 39.8272, 226.7124) (-29.4414, 39.8272, 216.2002) (-21.411, 39.8272, 208.4084) (0, 39.8272, 228.354) (21.0831, 39.8272, 226.7124) (29.4414, 39.8272, 216.2002) (21.411, 39.8272, 208.4084) (0, 39.8272, 180.975) (-19.2022, 39.8272, 182.0175) (-22.1651, 39.8272, 188.9101) (-31.8716, 39.8272, 192.9306) (-32.4063, 39.8272, 205.6433) (19.2022, 39.8272, 182.0175) (22.1651, 39.8272, 188.9101) (31.8716, 39.8272, 192.9306) (32.4063, 39.8272, 205.6433) on bodies 3
sketch "Sketch16" plane through (0, 0, 231.529) normal (0, 0, 1) x (1, 0, 0)
  line L0 (-12.7, 32.8422) -> (-12.7, 6.35)
  line L1 (-12.7, 6.35) -> (12.7, 6.35)
  line L2 (12.7, 6.35) -> (12.7, 32.8422)
  circle A0 centre (0, 24.7722) radius 3.2
  circle A1 centre (0, 24.7722) radius 6.4999
  line L3 (12.7, 32.8422) -> (-12.7, 32.8422)
  dimension "d140" = 12.9997
  constraint concentric A0 A1
  measures "d140" diameter of A1
extrude "Extrude16" cut sketch "Sketch16" against normal up to surface (3.175 mm away) contours A0 | A1 bodies 2
extrude "Extrude18" cut 4 faces at (-87.2067, 3.302, -152.8364) (-81.7033, 3.302, -152.8364) (81.7033, 3.302, -152.8364) (87.2067, 3.302, -152.8364) along direction (0, -1, 0) blind 1.016 on bodies 1 bodies 1
equation "d12 = outer_diameter"
equation "d13 = l1_mirror_base_h"
equation "d17 = l1_mirror_h"
equation "d18 = outer_diameter"
equation "d19 = mirror_diameter"
equation "d22 = l2_led_base_h"
equation "d23 = outer_diameter"
equation "d24 = led_base_inner_diameter"
equation "d27 = l2_led_h"
equation "d28 = outer_diameter"
equation "d29 = led_layer_inner_diameter"
equation "d32 = l3_glass_h"
equation "d33 = outer_diameter"
equation "d34 = mirror_diameter"
equation "d42 = l4_cap_height"
equation "d43 = outer_diameter"
equation "d91 = ( outer_diameter / 2 ) - ( screw_head_diameter / 2 ) - edge_tolerance"
equation "d99 = screw_head_diameter"
equation "d1 = ( 360 / ( 60 * 2 ) ) * 1 deg"
equation "d6 = led_base_inner_diameter"
equation "d7 = ( 360 / ( 60 * 2 ) ) * 1 deg"
equation "d10 = led_layer_inner_diameter - led_thickness"
equation "d124 = ( 3 / 64 ) * 1 in"
equation "l1_mirror_base_h = 0.13 in" comment "base layer thickness"
equation "l1_mirror_h = 0.12 in" comment "mirror thickness + tolerance"
equation "l2_led_base_h = 0.305 in" comment "mirror cap thickness"
equation "l2_led_h = 0.738 in" comment "LED layer thickness"
equation "l3_glass_h = 0.15 in" comment "glass layer thickness"
equation "l4_cap_height = 0.25 in" comment "top layer"
equation "outer_diameter = 14.25 in"
equation "edge_tolerance = 0.3 in"
equation "screw_head_diameter = 0.35 in"
equation "led_layer_inner_diameter = 12.57 in"
equation "led_base_inner_diameter = 12 in"
equation "led_thickness = 0.2 in"
equation "mirror_diameter = 12.85 in"
named bodies: "layer_one_base", "layer_three_cap", "layer_two_leds"
